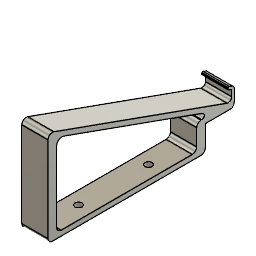
Laptop Stand 1 (Autodesk Fusion 360 design; units mm, degrees)
part number: 2025-09-20-18-01-36-899
Autodesk Fusion 360 part; units mm, degrees
sketch "Sketch5" plane through (0, 0, 0) normal (0, 1, 0) x (1, 0, 0)
  line L0 (0, 0) -> (-30, 0)
  line L1 (-30, 0) -> (-30, -180)
  line L2 (-30, -180) -> (0, -180)
  line L3 (0, -180) -> (0, 0)
  dimension "d12" = 30
  dimension "d13" = 180
  constraint horizontal L0
  constraint vertical L1
  constraint horizontal L2
  constraint vertical L3
  constraint coincident L0.start L3.end
  measures "d12" distance of L0.start L0.end
  measures "d13" distance of L0.start L2.end
extrude "Extrude4" add sketch "Sketch5" along normal blind 4
sketch "Sketch6" plane through (0, 4, 0) normal (0, 1, 0) x (-1, 0, 0)
  line L0 (0, 180) -> (0, 0)
  line L1 (0, 0) -> (30, 0)
  line L2 (30, 0) -> (30, 180)
  line L3 (30, 180) -> (0, 180)
  line L4 (0, 180) -> (30, 180)
  line L5 (30, 180) -> (30, 170)
  line L6 (30, 170) -> (0, 170)
  line L7 (0, 170) -> (0, 180)
  dimension "d16" = 10
  constraint horizontal L4
  constraint vertical L5
  constraint horizontal L6
  constraint vertical L7
  constraint coincident L2 L5.end
  constraint coincident L0.start L3.end
  measures "d16" distance of L0.start L6.end
extrude "Extrude5" add sketch "Sketch6" along normal blind 106 contours L0 L2 L3 L4 L5 L6 L7
sketch "Sketch7" plane through (0, 4, 0) normal (0, 1, 0) x (-1, 0, 0)
  line L0 (30, 170) -> (0, 170)
  line L1 (0, 170) -> (0, 0)
  line L2 (0, 0) -> (30, 0)
  line L3 (30, 0) -> (30, 170)
  line L4 (0, 0) -> (30, 0)
  line L5 (30, 0) -> (30, 10)
  line L6 (30, 10) -> (0, 10)
  line L7 (0, 10) -> (0, 0)
  dimension "d19" = 10
  constraint horizontal L4
  constraint vertical L5
  constraint horizontal L6
  constraint vertical L7
  constraint coincident L1.end L2.start
  measures "d19" distance of L1.end L6.end
extrude "Extrude6" add sketch "Sketch7" along normal blind 25 contours L1 L2 L3 L4 L5 L6 L7
sketch "Sketch8" plane through (-30, 0, 0) normal (-1, 0, 0) x (0, 0, 1)
  line L0 (0, 0) -> (180, 0)
  line L1 (180, 0) -> (180, 110)
  line L2 (180, 110) -> (170, 110)
  line L3 (170, 110) -> (170, 4)
  line L4 (170, 4) -> (10, 4)
  line L5 (10, 4) -> (10, 29)
  line L6 (10, 29) -> (0, 29)
  line L7 (0, 29) -> (0, 0)
  line L8 (10, 29) -> (-30, 29)
  line L9 (-30, 29) -> (-30, 35)
  line L10 (-30, 35) -> (10, 35)
  line L11 (10, 35) -> (10, 29)
  dimension "d22" = 40
  dimension "d23" = 6
  constraint horizontal L8
  constraint vertical L9
  constraint horizontal L10
  constraint vertical L11
  constraint coincident L5.end L6.start
  measures "d22" distance of L5.end L8.end
  measures "d23" distance of L5.end L10.end
extrude "Extrude7" add sketch "Sketch8" against normal blind 30 contours L6 L8 L9 L10 L11
sketch "Sketch9" plane through (-30, 0, 0) normal (-1, 0, 0) x (0, 0, 1)
  line L0 (0, 0) -> (180, 0)
  line L1 (180, 0) -> (180, 110)
  line L2 (180, 110) -> (170, 110)
  line L3 (170, 110) -> (170, 4)
  line L4 (170, 4) -> (10, 4)
  line L5 (10, 4) -> (10, 35)
  line L6 (10, 35) -> (-30, 35)
  line L7 (-30, 35) -> (-30, 29)
  line L8 (-30, 29) -> (0, 29)
  line L9 (0, 29) -> (0, 0)
  line L10 (-30, 35) -> (180, 110)
  line L11 (-30, 29) -> (180, 104)
  line L12 (180, 104) -> (180, 110)
  line L13 (-30, 35) -> (-30, 29)
  constraint coincident L6.end L7.start
  constraint coincident L1.end L2.start
  constraint coincident L7.end L8.start
  constraint coincident L1 L11.end
  constraint parallel L10 L11
extrude "Extrude8" add sketch "Sketch9" against normal blind 30 contours L3 L6 L10 L11
sketch "Sketch10" plane through (-30, 0, 0) normal (-1, 0, 0) x (0, 0, 1)
  line L0 (170, 100.4286) -> (170, 4)
  line L1 (170, 4) -> (10, 4)
  line L2 (10, 4) -> (10, 35)
  line L3 (10, 35) -> (-13.2, 35)
  line L4 (-13.2, 35) -> (170, 100.4286)
  line L5 (170, 106.4286) -> (-30, 35)
  line L6 (-30, 35) -> (-30, 29)
  line L7 (-30, 29) -> (0, 29)
  line L8 (0, 29) -> (0, 0)
  line L9 (0, 0) -> (180, 0)
  line L10 (180, 0) -> (180, 110)
  line L11 (180, 110) -> (170, 110)
  line L12 (170, 110) -> (170, 106.4286)
  line L13 (180, 110) -> (170, 106.4286)
  line L14 (170, 110) -> (180, 110)
  constraint coincident L10.end L11.start
  constraint coincident L5.start L12.end
  constraint coincident L11.end L12.start
extrude "Extrude9" cut sketch "Sketch10" against normal blind 30 contours L11 L12 L13 L14
extrude "Extrude10" add 1 faces at (-20, 4, 63.3333) along direction (0, 1, 0) blind 2
sketch "Sketch11" plane through (-30, 0, 0) normal (-1, 0, 0) x (0, 0, 1)
  line L0 (180, 110) -> (-30, 35)
  line L1 (-30, 35) -> (-30, 29)
  line L2 (-30, 29) -> (0, 29)
  line L3 (0, 29) -> (0, 0)
  line L4 (0, 0) -> (180, 0)
  line L5 (180, 0) -> (180, 110)
  line L6 (170, 6) -> (10, 6)
  line L7 (10, 6) -> (10, 35)
  line L8 (10, 35) -> (-13.2, 35)
  line L9 (-13.2, 35) -> (170, 100.4286)
  line L10 (170, 100.4286) -> (170, 6)
  line L11 (-30, 29) -> (-33, 29)
  line L12 (-33, 29) -> (-33, 48)
  line L13 (-33, 48) -> (-30, 48)
  line L14 (-30, 48) -> (-30, 29)
  dimension "d32" = 3
  dimension "d33" = 19
  constraint horizontal L11
  constraint vertical L12
  constraint horizontal L13
  constraint vertical L14
  constraint coincident L1.end L2.start
  measures "d32" distance of L1.end L11.end
  measures "d33" distance of L1.end L13.end
extrude "Extrude11" add sketch "Sketch11" against normal blind 30 contours L1 L11 L12 L13 L14
sketch "Sketch12" plane through (-30, 0, 0) normal (-1, 0, 0) x (0, 0, 1)
  line L0 (180, 110) -> (-30, 35)
  line L1 (-30, 35) -> (-30, 48)
  line L2 (-30, 48) -> (-33, 48)
  line L3 (-33, 48) -> (-33, 29)
  line L4 (-33, 29) -> (0, 29)
  line L5 (0, 29) -> (0, 0)
  line L6 (0, 0) -> (180, 0)
  line L7 (180, 0) -> (180, 110)
  line L8 (170, 6) -> (10, 6)
  line L9 (10, 6) -> (10, 35)
  line L10 (10, 35) -> (-13.2, 35)
  line L11 (-13.2, 35) -> (170, 100.4286)
  line L12 (170, 100.4286) -> (170, 6)
  line L13 (-30, 48) -> (-25.2926, 49.6855)
  line L14 (-30, 48) -> (-25, 48) construction
  line L15 (-25.2926, 49.6855) -> (-26.3039, 52.5099)
  line L16 (-26.3039, 52.5099) -> (-33, 50.1123)
  line L17 (-33, 50.1123) -> (-33, 48)
  dimension "d38" = 5
  dimension "d39" = 19.7
  dimension "d40" = 3
  constraint horizontal L14
  constraint coincident L1.end L2.start
  constraint perpendicular L13 L15
  constraint perpendicular L15 L16
  constraint coincident L2.end L3.start
  constraint perpendicular L2 L17
  measures "d38" distance of L1.end L13.end
  measures "d39" angle of L13 L14
  measures "d40" distance of L13.end L15.end
extrude "Extrude12" add sketch "Sketch12" against normal blind 30 contours L2 L13 L15 L16 L17
fillet "Fillet1" radius 5 1 edges at (-15, 29, -33)
fillet "Fillet2" radius 3 1 edges at (-15, 50.1123, -33)
fillet "Fillet3" radius 4 1 edges at (-15, 35, -30)
fillet "Fillet4" radius 1 2 edges at (-15, 52.5099, -26.3039) (-15, 49.6855, -25.2926)
fillet "Fillet5" radius 2 1 edges at (-15, 35, -13.2)
fillet "Fillet6" radius 5 1 edges at (-15, 110, 180)
fillet "Fillet7" radius 5 2 edges at (-15, 0, 0) (-15, 0, 180)
fillet "Fillet8" radius 5 4 edges at (-15, 35, 10) (-15, 6, 10) (-15, 100.4286, 170) (-15, 6, 170)
sketch "Sketch13" plane through (0, 6, 0) normal (0, 1, 0) x (-1, 0, 0)
  line L0 (30, 165) -> (0, 165)
  line L1 (0, 165) -> (0, 15)
  line L2 (0, 15) -> (30, 15)
  line L3 (30, 15) -> (30, 165)
  circle A0 centre (15, 50) radius 4
  circle A1 centre (15, 130) radius 4
  dimension "d59" = 8
  dimension "d61" = 8
  dimension "d62" = 80
  dimension "d63" = 35
  measures "d59" diameter of A0
  measures "d61" diameter of A1
  measures "d62" distance of A0.centre A1.centre
  measures "d63" distance of L0 A1.centre
extrude "Extrude13" cut sketch "Sketch13" against normal blind 6 contours A0 | A1
delete_face "DeleteFace1" 1 faces at (-20, 36.0576, -3.4176)
fillet "Fillet9" radius 3 1 edges at (-15, 35, -13.2)
delete_face "DeleteFace2" 1 faces at (-20, 98.2371, 165.9775)
fillet "Fillet10" radius 6 1 edges at (-15, 100.4286, 170)
